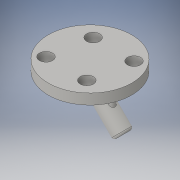
# Autodesk Inventor part: motor_mount
Saved by Autodesk Inventor 2016 (Build 200138000, 138)
## iProperties
Created: 2016-03-06
Part Number: motor_mount
Material: Generic
Document SubType Name: Modeling
Designer: dimas
Density: 1 g/cm^3
Appearance: Default
Author: dimas
Autodesk Inventor part; units mm, degrees
ref_plane "YZ Plane" through (0, 0, 0) normal (1, 0, 0) x (0, 1, 0)
ref_plane "XZ Plane" through (0, 0, 0) normal (0, 1, 0) x (-1, 0, 0)
ref_plane "XY Plane" through (0, 0, 0) normal (0, 0, 1) x (1, 0, 0)
sketch "Sketch1" plane through (0, 0, 0) normal (0, 1, 0) x (-1, 0, 0)
  circle A0 centre (0, 0) radius 9.5
  circle A1 centre (0, 0) radius 8
  circle A2 centre (0, 0) radius 12.7
  dimension "d0" = 19
  dimension "d1" = 16
  dimension "d2" = 25.4
  constraints: 3 centre point, 3 coincident
  measures "d0" diameter of A0
  measures "d1" diameter of A1
  measures "d2" diameter of A2
extrude "Extrusion1" add sketch "Sketch1" along normal blind 3.175 contours A0 | A1 | A2
sketch "Sketch2" plane through (0, 3.175, 0) normal (0, 1, 0) x (1, 0, 0)
  circle A0 centre (0, 0) radius 8
  circle A1 centre (0, 0) radius 9.5
  line L0 (0, 0) -> (0, -6.1214)
  line L1 (0, -6.1214) -> (5.1506, -6.1214)
  line L2 (0, -6.1214) -> (-7.2649, -6.1214)
  line L3 (0, 0) -> (0, 6.1214)
  line L4 (0, 6.1214) -> (-5.1506, 6.1214)
  line L5 (0, 6.1214) -> (7.2649, 6.1214)
  dimension "d5" = 16
  dimension "d6" = 19
  dimension "d7" = 6.1214
  dimension "d8" = 6.1214
  constraints: 12 end point, 4 point on circle, 2 centre point, 2 coincident, 2 point on line, 2 vertical, 1 horizontal, 1 perpendicular
  measures "d5" diameter of A0
  measures "d6" diameter of A1
  measures "d7" distance of L0.start L0.end
  measures "d8" distance of L0.start L3.end
hole "Hole1" at (-7.2649, 3.175, 6.1214) at (-5.1506, 3.175, -6.1214) at (7.2649, 3.175, -6.1214) at (5.1506, 3.175, 6.1214) direction (0, -1, 0) diameter 4 end through all
sketch "Sketch3" plane through (0, 0, 0) normal (0, -1, 0) x (1, 0, 0)
  line L0 (0, 0) -> (3.81, 0)
  line L1 (3.81, 0) -> (3.81, 3.81)
  line L2 (3.81, 3.81) -> (-3.81, 3.81)
  line L3 (-3.81, 3.81) -> (-3.81, -3.81)
  line L4 (-3.81, -3.81) -> (3.81, -3.81)
  line L5 (3.81, -3.81) -> (3.81, 3.81)
  dimension "d16" = 3.81
  dimension "d17" = 3.81
  dimension "d18" = 7.62
  dimension "d19" = 7.62
  constraints: 12 end point, 2 horizontal, 2 parallel, 2 perpendicular
  measures "d16" distance of L0.start L0.end
  measures "d17" distance of L0.end L1.end
  measures "d18" distance of L4.end L3.end
  measures "d19" distance of L3.end L2.end
extrude "Extrusion2" add sketch "Sketch3" along normal blind 7.62
sketch "Sketch5" plane through (-3.81, 0, 3.81) normal (0, 0, 1) x (1, 0, 0)
  line L0 (0, 0) -> (0, -7.62) projected
  line L1 (7.62, 0) -> (0, 0) projected
  line L2 (0, -7.62) -> (7.62, 0)
  line L3 (7.62, 0) -> (7.62, -7.62) projected
  line L4 (7.62, 0) -> (7.62, -7.62)
  line L5 (7.62, -7.62) -> (0, -7.62)
  point P0 (3.81, 0)
  constraints: 6 end point, 1 collinear, 1 perpendicular
extrude "Extrusion3" cut sketch "Sketch5" against normal blind 7.62 contours L2 L3 L5
sketch "Sketch6" plane through (-3.81, -7.62, 3.81) normal (0.7071068, -0.7071068, 0) x (-0.7071068, -0.7071068, 0)
  line L0 (-5.3882, 0) -> (-10.7763, 0) projected
  line L1 (-10.7763, 0) -> (-3.1563, 0)
  line L2 (-10.7763, 7.62) -> (-5.3882, 7.62) projected
  line L3 (-3.1563, 0) -> (-10.7763, 7.62)
  line L4 (-10.7763, 7.62) -> (-3.1563, 7.62)
  line L5 (-3.1563, 7.62) -> (-10.7763, 0)
  circle A0 centre (-6.9663, 3.81) radius 2.5
  point P0 (-8.0822, 3.81)
  dimension "d24" = 7.62
  dimension "d25" = 5
  constraints: 8 end point, 1 centre point, 1 collinear, 1 midpoint, 1 parallel, 1 perpendicular
  measures "d24" distance of L0.end L1.end
  measures "d25" diameter of A0
extrude "Extrusion4" add sketch "Sketch6" along normal blind 12.7 contours A0 L3 L5 | L5 L3 A0 | L3 L5 A0 | L3 A0 L5
sketch "Sketch7" plane through (-3.81, -7.62, 3.81) normal (0.7071068, -0.7071068, 0) x (-0.7071068, -0.7071068, 0)
  line L0 (-10.7763, 0) -> (-10.7763, 7.62) projected
  line L1 (-5.3882, 0) -> (0, 0) projected
  line L2 (-10.7763, 7.62) -> (0, 7.62)
  line L3 (0, 7.62) -> (0, 0)
  line L4 (0, 0) -> (-10.7763, 0)
  line L5 (-10.7763, 0) -> (-10.7763, 7.62)
  circle A0 centre (-6.9663, 3.81) radius 2.5 projected
  circle A1 centre (-6.9663, 3.81) radius 2.5
  point P0 (-8.0822, 3.81)
  constraints: 8 end point, 2 parallel, 1 centre point, 1 coincident, 1 horizontal, 1 perpendicular
sketch "Sketch8" plane through (-3.81, 0, -3.81) normal (-1, 0, 0) x (0, 0, 1)
  line L0 (7.62, -7.62) -> (0, -7.62) projected
  line L1 (0, 0) -> (0, -7.62) projected
  line L2 (7.62, -7.62) -> (0, -7.62)
  line L3 (0, -7.62) -> (0, 0)
  line L4 (0, 0) -> (7.62, 0)
  line L5 (7.62, 0) -> (7.62, -7.62)
  point P0 (3.81, 0)
  constraints: 8 end point, 2 parallel, 1 horizontal, 1 perpendicular
extrude "Extrusion5" add sketch "Sketch8" along normal blind 3.81
sketch "Sketch9" plane through (3.81, 0, -3.81) normal (0, 0, -1) x (-1, 0, 0)
  line L0 (7.62, -7.62) -> (11.43, -3.81)
  line L1 (11.43, 0) -> (11.43, -7.62) projected
  line L2 (11.43, -7.62) -> (11.43, -3.81)
  line L3 (11.43, -7.62) -> (7.62, -7.62)
  point P0 (3.81, 0)
  constraints: 6 end point, 1 collinear, 1 midpoint, 1 perpendicular
extrude "Extrusion6" cut sketch "Sketch9" against normal through all
extrude "Extrusion7" cut sketch "Sketch7" against normal up to surface surface through (0, 0, 0) normal (0, 1, 0)
sketch "Sketch10" plane through (10.0962, -11.6743, 0) normal (0.7071068, -0.7071068, 0) x (-0.7071068, -0.7071068, 0)
  circle A0 centre (0, 0) radius 1.5
  point P0 (-1.1159, 0)
  dimension "d34" = 3
  constraints: 1 centre point
  measures "d34" diameter of A0
extrude "Extrusion8" cut sketch "Sketch10" against normal blind 12.7
fillet "Fillet1" radius 0.635 1 edges at (11.8639, -9.9066, 0)
fillet "Fillet2" radius 0.508 1 edges at (11.1568, -10.6137, 0)
sketch "Sketch11" plane through (0, 0, 0) normal (0, -1, 0) x (1, 0, 0)
  line L0 (0, 0) -> (7.62, 0)
  line L1 (7.62, 0) -> (7.62, -1)
  line L2 (7.62, -1) -> (0, -1)
  line L3 (0, -1) -> (0, 1.032)
  line L4 (0, 1.032) -> (7.62, 1.032)
  line L5 (7.62, 1.032) -> (7.62, -1)
  dimension "d39" = 7.62
  dimension "d40" = 1
  dimension "d41" = 7.62
  dimension "d42" = 2.032
  constraints: 12 end point, 2 horizontal, 2 parallel, 1 perpendicular, 1 vertical
  measures "d39" distance of L0.start L0.end
  measures "d40" distance of L0.end L1.end
  measures "d41" distance of L3.end L4.end
  measures "d42" distance of L2.end L3.end
extrude "Extrusion9" add sketch "Sketch11" along normal up to surface round surface about axis through (1.1159, -2.6941, 0) along (0.7071068, -0.7071068, 0) radius 2.5 far side no
extrude "Extrusion10" cut sketch "Sketch10" against normal blind 12.7
full round fillet "Fillet3" first side at (5.6341, -1.9859, -1) centre faces at (7.62, -1.8899, -0.0424) second side at (5.6274, -1.9926, 1.032)
body "Solid1"
